Autodesk Fusion 360 part; units mm, degrees
note: some values were not read from the file. Set by a fixed rule: which sketch regions a step uses.
(part 14 of 14)
  spline S78 degree 5 poles (-18.9704, 3.8829) (-18.9704, 3.8829) (-18.9706, 3.883) (-18.9708, 3.883) (-18.9712, 3.8831) (-18.9718, 3.8832) (-18.9725, 3.8833) (-18.9733, 3.8835) (-18.9742, 3.8836) (-18.9751, 3.8838) (-18.9761, 3.884) (-18.9773, 3.8842) (-18.9785, 3.8844) (-18.9798, 3.8846) (-18.9811, 3.8848) (-18.9826, 3.8851) (-18.9841, 3.8853) (-18.9858, 3.8856) (-18.9875, 3.8859) (-18.9892, 3.8862) (-18.9911, 3.8865) (-18.993, 3.8868) (-18.9951, 3.8871) (-18.9972, 3.8874) (-18.9993, 3.8877) (-19.0016, 3.888) (-19.0039, 3.8884) (-19.0063, 3.8887) (-19.0088, 3.889) (-19.0113, 3.8894) (-19.0139, 3.8898) (-19.0166, 3.8901) (-19.0194, 3.8905) (-19.0222, 3.8908) (-19.0251, 3.8912) (-19.0281, 3.8916) (-19.0311, 3.892) (-19.0342, 3.8923) (-19.0374, 3.8927) (-19.0406, 3.8931) (-19.0439, 3.8935) (-19.0473, 3.8939) (-19.0507, 3.8942) (-19.0542, 3.8946) (-19.0578, 3.895) (-19.0615, 3.8954) (-19.0652, 3.8958) (-19.0689, 3.8962) (-19.0727, 3.8965) (-19.0766, 3.8969) (-19.0806, 3.8973) (-19.0846, 3.8977) (-19.0887, 3.898) (-19.0928, 3.8984) (-19.097, 3.8988) (-19.1013, 3.8992) (-19.1056, 3.8995) (-19.11, 3.8999) (-19.1144, 3.9002) (-19.1189, 3.9006) (-19.1235, 3.9009) (-19.1281, 3.9013) (-19.1327, 3.9016) (-19.1375, 3.902) (-19.1423, 3.9023) (-19.1471, 3.9026) (-19.152, 3.9029) (-19.157, 3.9032) (-19.162, 3.9035) (-19.167, 3.9039) (-19.1721, 3.9041) (-19.1773, 3.9044) (-19.1825, 3.9047) (-19.1878, 3.905) (-19.1932, 3.9053) (-19.1985, 3.9055) (-19.204, 3.9058) (-19.2095, 3.906) (-19.215, 3.9063) (-19.2206, 3.9065) (-19.2263, 3.9067) (-19.232, 3.9069) (-19.2377, 3.9071) (-19.2435, 3.9073) (-19.2494, 3.9075) (-19.2553, 3.9077) (-19.2612, 3.9079) (-19.2672, 3.908) (-19.2733, 3.9082) (-19.2794, 3.9083) (-19.2855, 3.9085) (-19.2917, 3.9086) (-19.2979, 3.9087) (-19.3042, 3.9088) (-19.3106, 3.9089) (-19.317, 3.909) (-19.3234, 3.9091) (-19.3299, 3.9091) (-19.3364, 3.9092) (-19.343, 3.9092) (-19.3496, 3.9093) (-19.3563, 3.9093) (-19.363, 3.9093) (-19.3697, 3.9093) (-19.3765, 3.9093) (-19.3834, 3.9092) (-19.3903, 3.9092) (-19.3972, 3.9091) (-19.4042, 3.9091) (-19.4112, 3.909) (-19.4183, 3.9089) (-19.4254, 3.9088) (-19.4325, 3.9087) (-19.4397, 3.9085) (-19.447, 3.9084) (-19.4542, 3.9082) (-19.4616, 3.9081) (-19.4689, 3.9079) (-19.4763, 3.9077) (-19.4838, 3.9075) (-19.4913, 3.9073) (-19.4988, 3.907) (-19.5064, 3.9068) (-19.514, 3.9065) (-19.5216, 3.9062) (-19.5293, 3.9059) (-19.5371, 3.9056) (-19.5448, 3.9053) (-19.5527, 3.905) (-19.5605, 3.9046) (-19.5684, 3.9043) (-19.5763, 3.9039) (-19.5843, 3.9035) (-19.5923, 3.9031) (-19.6004, 3.9027) (-19.6085, 3.9022) (-19.6166, 3.9018) (-19.6248, 3.9013) (-19.633, 3.9008) (-19.6412, 3.9003) (-19.6495, 3.8998) (-19.6578, 3.8992) (-19.6661, 3.8987) (-19.6745, 3.8981) (-19.683, 3.8975) (-19.6914, 3.8969) (-19.6999, 3.8963) (-19.7084, 3.8957) (-19.717, 3.8951) (-19.7256, 3.8944) (-19.7343, 3.8937) (-19.7429, 3.893) (-19.7517, 3.8923) (-19.7604, 3.8916) (-19.7692, 3.8908) (-19.778, 3.89) (-19.7869, 3.8893) (-19.7958, 3.8885) (-19.8047, 3.8876) (-19.8136, 3.8868) (-19.8226, 3.886) (-19.8317, 3.8851) (-19.8407, 3.8842) (-19.8498, 3.8833) (-19.8589, 3.8824) (-19.8681, 3.8814) (-19.8773, 3.8805) (-19.8865, 3.8795) (-19.8958, 3.8785) (-19.9051, 3.8775) (-19.9144, 3.8765) (-19.9237, 3.8754) (-19.9331, 3.8743) (-19.9426, 3.8733) (-19.952, 3.8722) (-19.9615, 3.871) (-19.971, 3.8699) (-19.9806, 3.8687) (-19.9901, 3.8675) (-19.9997, 3.8663) (-20.0094, 3.8651) (-20.0191, 3.8639) (-20.0288, 3.8626) (-20.0385, 3.8614) (-20.0483, 3.8601) (-20.0581, 3.8588) (-20.0679, 3.8574) (-20.0777, 3.8561) (-20.0876, 3.8547) (-20.0975, 3.8533) (-20.1075, 3.8519) (-20.1175, 3.8505) (-20.1275, 3.849) (-20.1375, 3.8476) (-20.1476, 3.8461) (-20.1577, 3.8446) (-20.1678, 3.843) (-20.1779, 3.8415) (-20.1881, 3.8399) (-20.1983, 3.8383) (-20.2085, 3.8367) (-20.2188, 3.8351) (-20.2291, 3.8334) (-20.2394, 3.8318) (-20.2498, 3.8301) (-20.2601, 3.8284) (-20.2705, 3.8267) (-20.281, 3.8249) (-20.2914, 3.8231) (-20.3019, 3.8213) (-20.3124, 3.8195) (-20.323, 3.8177) (-20.3335, 3.8158) (-20.3441, 3.814) (-20.3547, 3.8121) (-20.3654, 3.8102) (-20.3761, 3.8082) (-20.3868, 3.8063) (-20.3975, 3.8043) (-20.4082, 3.8023) (-20.419, 3.8003) (-20.4298, 3.7982) (-20.4406, 3.7962) (-20.4515, 3.7941) (-20.4624, 3.792) (-20.4733, 3.7898) (-20.4842, 3.7877) (-20.4952, 3.7855) (-20.5061, 3.7833) (-20.5171, 3.7811) (-20.5282, 3.7789) (-20.5392, 3.7766) (-20.5503, 3.7743) (-20.5614, 3.772) (-20.5725, 3.7697) (-20.5837, 3.7674) (-20.5948, 3.765) (-20.606, 3.7626) (-20.6173, 3.7602) (-20.6285, 3.7578) (-20.6398, 3.7553) (-20.6488, 3.7533) (-20.6556, 3.7519) (-20.6601, 3.7508) (-20.6624, 3.7503) knots 0 0 0 0 0 0 0.00416667 0.00833333 0.0125 0.01666667 0.02083333 0.025 0.02916667 0.03333333 0.0375 0.04166667 0.04583333 0.05 0.05416667 0.05833333 0.0625 0.06666667 0.07083333 0.075 0.07916667 0.08333333 0.0875 0.09166667 0.09583333 0.1 0.10416667 0.10833333 0.1125 0.11666667 0.12083333 0.125 0.12916667 0.13333333 0.1375 0.14166667 0.14583333 0.15 0.15416667 0.15833333 0.1625 0.16666667 0.17083333 0.175 0.17916667 0.18333333 0.1875 0.19166667 0.19583333 0.2 0.20416667 0.20833333 0.2125 0.21666667 0.22083333 0.225 0.22916667 0.23333333 0.2375 0.24166667 0.24583333 0.25 0.25416667 0.25833333 0.2625 0.26666667 0.27083333 0.275 0.27916667 0.28333333 0.2875 0.29166667 0.29583333 0.3 0.30416667 0.30833333 0.3125 0.31666667 0.32083333 0.325 0.32916667 0.33333333 0.3375 0.34166667 0.34583333 0.35 0.35416667 0.35833333 0.3625 0.36666667 0.37083333 0.375 0.37916667 0.38333333 0.3875 0.39166667 0.39583333 0.4 0.40416667 0.40833333 0.4125 0.41666667 0.42083333 0.425 0.42916667 0.43333333 0.4375 0.44166667 0.44583333 0.45 0.45416667 0.45833333 0.4625 0.46666667 0.47083333 0.475 0.47916667 0.48333333 0.4875 0.49166667 0.49583333 0.5 0.50416667 0.50833333 0.5125 0.51666667 0.52083333 0.525 0.52916667 0.53333333 0.5375 0.54166667 0.54583333 0.55 0.55416667 0.55833333 0.5625 0.56666667 0.57083333 0.575 0.57916667 0.58333333 0.5875 0.59166667 0.59583333 0.6 0.60416667 0.60833333 0.6125 0.61666667 0.62083333 0.625 0.62916667 0.63333333 0.6375 0.64166667 0.64583333 0.65 0.65416667 0.65833333 0.6625 0.66666667 0.67083333 0.675 0.67916667 0.68333333 0.6875 0.69166667 0.69583333 0.7 0.70416667 0.70833333 0.7125 0.71666667 0.72083333 0.725 0.72916667 0.73333333 0.7375 0.74166667 0.74583333 0.75 0.75416667 0.75833333 0.7625 0.76666667 0.77083333 0.775 0.77916667 0.78333333 0.7875 0.79166667 0.79583333 0.8 0.80416667 0.80833333 0.8125 0.81666667 0.82083333 0.825 0.82916667 0.83333333 0.8375 0.84166667 0.84583333 0.85 0.85416667 0.85833333 0.8625 0.86666667 0.87083333 0.875 0.87916667 0.88333333 0.8875 0.89166667 0.89583333 0.9 0.90416667 0.90833333 0.9125 0.91666667 0.92083333 0.925 0.92916667 0.93333333 0.9375 0.94166667 0.94583333 0.95 0.95416667 0.95833333 0.9625 0.96666667 0.97083333 0.975 0.97916667 0.98333333 0.9875 0.99166667 0.99583333 1 1 1 1 1 1
  arc A79 (-20.6624, 3.7503) -> (-20.81, 2.8182) centre (0, 0) ccw
  spline S79 degree 5 poles (-20.81, 2.8182) (-20.808, 2.8171) (-20.804, 2.8147) (-20.798, 2.8112) (-20.7901, 2.8065) (-20.7801, 2.8007) (-20.7702, 2.7949) (-20.7602, 2.7892) (-20.7503, 2.7834) (-20.7404, 2.7777) (-20.7305, 2.772) (-20.7207, 2.7664) (-20.7108, 2.7608) (-20.701, 2.7552) (-20.6912, 2.7496) (-20.6814, 2.7441) (-20.6716, 2.7386) (-20.6618, 2.7331) (-20.6521, 2.7277) (-20.6424, 2.7222) (-20.6326, 2.7168) (-20.6229, 2.7115) (-20.6133, 2.7061) (-20.6036, 2.7008) (-20.594, 2.6956) (-20.5843, 2.6903) (-20.5747, 2.6851) (-20.5652, 2.6799) (-20.5556, 2.6747) (-20.546, 2.6696) (-20.5365, 2.6645) (-20.527, 2.6594) (-20.5175, 2.6543) (-20.508, 2.6493) (-20.4986, 2.6443) (-20.4891, 2.6393) (-20.4797, 2.6344) (-20.4703, 2.6295) (-20.4609, 2.6246) (-20.4516, 2.6197) (-20.4422, 2.6149) (-20.4329, 2.6101) (-20.4236, 2.6053) (-20.4143, 2.6006) (-20.4051, 2.5958) (-20.3958, 2.5912) (-20.3866, 2.5865) (-20.3774, 2.5818) (-20.3683, 2.5772) (-20.3591, 2.5727) (-20.35, 2.5681) (-20.3409, 2.5636) (-20.3318, 2.5591) (-20.3227, 2.5546) (-20.3137, 2.5502) (-20.3046, 2.5458) (-20.2956, 2.5414) (-20.2867, 2.537) (-20.2777, 2.5327) (-20.2688, 2.5284) (-20.2599, 2.5241) (-20.251, 2.5199) (-20.2421, 2.5156) (-20.2333, 2.5114) (-20.2245, 2.5073) (-20.2157, 2.5031) (-20.2069, 2.499) (-20.1981, 2.495) (-20.1894, 2.4909) (-20.1807, 2.4869) (-20.172, 2.4829) (-20.1634, 2.4789) (-20.1548, 2.475) (-20.1462, 2.471) (-20.1376, 2.4672) (-20.1291, 2.4633) (-20.1205, 2.4595) (-20.112, 2.4557) (-20.1036, 2.4519) (-20.0951, 2.4481) (-20.0867, 2.4444) (-20.0783, 2.4407) (-20.0699, 2.437) (-20.0616, 2.4334) (-20.0533, 2.4298) (-20.045, 2.4262) (-20.0367, 2.4226) (-20.0285, 2.4191) (-20.0203, 2.4156) (-20.0121, 2.4121) (-20.0039, 2.4086) (-19.9958, 2.4052) (-19.9877, 2.4018) (-19.9797, 2.3984) (-19.9716, 2.3951) (-19.9636, 2.3918) (-19.9556, 2.3885) (-19.9477, 2.3852) (-19.9398, 2.382) (-19.9319, 2.3788) (-19.924, 2.3756) (-19.9162, 2.3724) (-19.9084, 2.3693) (-19.9006, 2.3662) (-19.8929, 2.3631) (-19.8851, 2.3601) (-19.8775, 2.357) (-19.8698, 2.354) (-19.8622, 2.3511) (-19.8546, 2.3481) (-19.847, 2.3452) (-19.8395, 2.3423) (-19.832, 2.3394) (-19.8246, 2.3366) (-19.8171, 2.3338) (-19.8098, 2.331) (-19.8024, 2.3282) (-19.7951, 2.3255) (-19.7878, 2.3228) (-19.7805, 2.3201) (-19.7733, 2.3175) (-19.7661, 2.3148) (-19.7589, 2.3122) (-19.7518, 2.3097) (-19.7447, 2.3071) (-19.7377, 2.3046) (-19.7306, 2.3021) (-19.7237, 2.2996) (-19.7167, 2.2971) (-19.7098, 2.2947) (-19.7029, 2.2923) (-19.6961, 2.29) (-19.6893, 2.2876) (-19.6825, 2.2853) (-19.6758, 2.283) (-19.6691, 2.2807) (-19.6624, 2.2785) (-19.6558, 2.2763) (-19.6492, 2.2741) (-19.6427, 2.2719) (-19.6362, 2.2698) (-19.6297, 2.2676) (-19.6233, 2.2655) (-19.6169, 2.2635) (-19.6106, 2.2614) (-19.6043, 2.2594) (-19.598, 2.2574) (-19.5918, 2.2555) (-19.5856, 2.2535) (-19.5795, 2.2516) (-19.5734, 2.2497) (-19.5673, 2.2478) (-19.5613, 2.246) (-19.5553, 2.2442) (-19.5494, 2.2424) (-19.5435, 2.2406) (-19.5377, 2.2388) (-19.5319, 2.2371) (-19.5261, 2.2354) (-19.5204, 2.2337) (-19.5147, 2.2321) (-19.5091, 2.2305) (-19.5035, 2.2289) (-19.498, 2.2273) (-19.4925, 2.2257) (-19.4871, 2.2242) (-19.4817, 2.2227) (-19.4763, 2.2212) (-19.471, 2.2197) (-19.4658, 2.2183) (-19.4606, 2.2169) (-19.4554, 2.2155) (-19.4503, 2.2141) (-19.4452, 2.2128) (-19.4402, 2.2115) (-19.4353, 2.2102) (-19.4304, 2.2089) (-19.4255, 2.2076) (-19.4207, 2.2064) (-19.4159, 2.2052) (-19.4112, 2.204) (-19.4066, 2.2028) (-19.402, 2.2017) (-19.3974, 2.2006) (-19.393, 2.1995) (-19.3885, 2.1984) (-19.3841, 2.1973) (-19.3798, 2.1963) (-19.3755, 2.1953) (-19.3713, 2.1943) (-19.3671, 2.1933) (-19.363, 2.1924) (-19.359, 2.1915) (-19.355, 2.1906) (-19.3511, 2.1897) (-19.3472, 2.1888) (-19.3434, 2.188) (-19.3396, 2.1872) (-19.3359, 2.1864) (-19.3323, 2.1856) (-19.3287, 2.1848) (-19.3252, 2.1841) (-19.3217, 2.1834) (-19.3183, 2.1827) (-19.315, 2.182) (-19.3117, 2.1813) (-19.3085, 2.1807) (-19.3054, 2.1801) (-19.3023, 2.1795) (-19.2993, 2.1789) (-19.2964, 2.1783) (-19.2935, 2.1778) (-19.2907, 2.1772) (-19.288, 2.1767) (-19.2853, 2.1762) (-19.2827, 2.1758) (-19.2802, 2.1753) (-19.2777, 2.1749) (-19.2753, 2.1745) (-19.273, 2.1741) (-19.2708, 2.1737) (-19.2686, 2.1733) (-19.2665, 2.173) (-19.2645, 2.1726) (-19.2626, 2.1723) (-19.2607, 2.172) (-19.259, 2.1718) (-19.2573, 2.1715) (-19.2556, 2.1712) (-19.2541, 2.171) (-19.2526, 2.1708) (-19.2512, 2.1706) (-19.2499, 2.1704) (-19.2487, 2.1702) (-19.2476, 2.1701) (-19.2466, 2.1699) (-19.2456, 2.1698) (-19.2447, 2.1697) (-19.244, 2.1696) (-19.2433, 2.1695) (-19.2427, 2.1694) (-19.2423, 2.1694) (-19.242, 2.1693) (-19.2418, 2.1693) (-19.2418, 2.1693) knots -1 -1 -1 -1 -1 -1 -0.99583333 -0.99166667 -0.9875 -0.98333333 -0.97916667 -0.975 -0.97083333 -0.96666667 -0.9625 -0.95833333 -0.95416667 -0.95 -0.94583333 -0.94166667 -0.9375 -0.93333333 -0.92916667 -0.925 -0.92083333 -0.91666667 -0.9125 -0.90833333 -0.90416667 -0.9 -0.89583333 -0.89166667 -0.8875 -0.88333333 -0.87916667 -0.875 -0.87083333 -0.86666667 -0.8625 -0.85833333 -0.85416667 -0.85 -0.84583333 -0.84166667 -0.8375 -0.83333333 -0.82916667 -0.825 -0.82083333 -0.81666667 -0.8125 -0.80833333 -0.80416667 -0.8 -0.79583333 -0.79166667 -0.7875 -0.78333333 -0.77916667 -0.775 -0.77083333 -0.76666667 -0.7625 -0.75833333 -0.75416667 -0.75 -0.74583333 -0.74166667 -0.7375 -0.73333333 -0.72916667 -0.725 -0.72083333 -0.71666667 -0.7125 -0.70833333 -0.70416667 -0.7 -0.69583333 -0.69166667 -0.6875 -0.68333333 -0.67916667 -0.675 -0.67083333 -0.66666667 -0.6625 -0.65833333 -0.65416667 -0.65 -0.64583333 -0.64166667 -0.6375 -0.63333333 -0.62916667 -0.625 -0.62083333 -0.61666667 -0.6125 -0.60833333 -0.60416667 -0.6 -0.59583333 -0.59166667 -0.5875 -0.58333333 -0.57916667 -0.575 -0.57083333 -0.56666667 -0.5625 -0.55833333 -0.55416667 -0.55 -0.54583333 -0.54166667 -0.5375 -0.53333333 -0.52916667 -0.525 -0.52083333 -0.51666667 -0.5125 -0.50833333 -0.50416667 -0.5 -0.49583333 -0.49166667 -0.4875 -0.48333333 -0.47916667 -0.475 -0.47083333 -0.46666667 -0.4625 -0.45833333 -0.45416667 -0.45 -0.44583333 -0.44166667 -0.4375 -0.43333333 -0.42916667 -0.425 -0.42083333 -0.41666667 -0.4125 -0.40833333 -0.40416667 -0.4 -0.39583333 -0.39166667 -0.3875 -0.38333333 -0.37916667 -0.375 -0.37083333 -0.36666667 -0.3625 -0.35833333 -0.35416667 -0.35 -0.34583333 -0.34166667 -0.3375 -0.33333333 -0.32916667 -0.325 -0.32083333 -0.31666667 -0.3125 -0.30833333 -0.30416667 -0.3 -0.29583333 -0.29166667 -0.2875 -0.28333333 -0.27916667 -0.275 -0.27083333 -0.26666667 -0.2625 -0.25833333 -0.25416667 -0.25 -0.24583333 -0.24166667 -0.2375 -0.23333333 -0.22916667 -0.225 -0.22083333 -0.21666667 -0.2125 -0.20833333 -0.20416667 -0.2 -0.19583333 -0.19166667 -0.1875 -0.18333333 -0.17916667 -0.175 -0.17083333 -0.16666667 -0.1625 -0.15833333 -0.15416667 -0.15 -0.14583333 -0.14166667 -0.1375 -0.13333333 -0.12916667 -0.125 -0.12083333 -0.11666667 -0.1125 -0.10833333 -0.10416667 -0.1 -0.09583333 -0.09166667 -0.0875 -0.08333333 -0.07916667 -0.075 -0.07083333 -0.06666667 -0.0625 -0.05833333 -0.05416667 -0.05 -0.04583333 -0.04166667 -0.0375 -0.03333333 -0.02916667 -0.025 -0.02083333 -0.01666667 -0.0125 -0.00833333 -0.00416667 0 0 0 0 0 0
  line L158 (-19.2418, 2.1693) -> (-19.2411, 2.1692)
  line L159 (-19.2411, 2.1692) -> (-18.632, 2.1005)
  circle A80 centre (0, 0) radius 2.65
  circle A81 centre (0, 0) radius 6
  circle A82 centre (0, -6) radius 1.15
  circle A83 centre (4.2426, -4.2426) radius 1.15
  circle A84 centre (6, 0) radius 1.15
  circle A85 centre (4.2426, 4.2426) radius 1.15
  circle A86 centre (0, 6) radius 1.15
  circle A87 centre (-4.2426, 4.2426) radius 1.15
  circle A88 centre (-6, 0) radius 1.15
  circle A89 centre (-4.2426, -4.2426) radius 1.15
  dimension "d7" = 5.3
  dimension "d8" = 12
  dimension "d9" = 2.3
  dimension "d11" = 360
  constraint coincident A0.centre A1.centre
  constraint coincident A81 A82.centre
  measures "d7" diameter of A80
  measures "d8" diameter of A81
  measures "d9" diameter of A82
extrude "돌출3" cut sketch "스케치1 (2)" against normal blind 9 contours A80 | A81 A84 | A81 A84 | A81 A85 | A81 A85 | A81 A83 | A81 A83 | A81 A86 | A81 A86 | A81 A82 | A81 A82 | A81 A87 | A81 A87 | A81 A89 | A81 A89 | A81 A88 | A81 A88 bodies 1 in component "Component"
component "Component" placed x (1, 0, 0) y (0, 1, 0) z (0, 0, 1) at (0, 0, 0)
